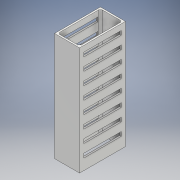
# Autodesk Inventor part: LiFeGuard
Saved by Autodesk Inventor 2018 (Build 220112000, 112)
## iProperties
Created: 2018-08-27
Part Number: LiFeGuard
Material: ABS プラスチック
Document SubType Name: Modeling
Designer: shun2
Density: 1.06 g/cm^3
Appearance: 滑らか - 白
Author: shun2
Autodesk Inventor part; units mm, degrees
ref_plane "YZ Plane" through (0, 0, 0) normal (1, 0, 0) x (0, 1, 0)
ref_plane "XZ Plane" through (0, 0, 0) normal (0, 1, 0) x (-1, 0, 0)
ref_plane "XY Plane" through (0, 0, 0) normal (0, 0, 1) x (1, 0, 0)
sketch "スケッチ1" plane through (0, 0, 0) normal (0, 0, 1) x (1, 0, 0)
  line L0 (0, 0) -> (30, 0)
  line L1 (30, 0) -> (30, 55)
  line L2 (30, 55) -> (0, 55)
  line L3 (0, 55) -> (0, 2)
  line L4 (2, 53) -> (2, 2)
  line L5 (2, 2) -> (28, 2)
  line L6 (28, 53) -> (28, 2)
  line L7 (2, 53) -> (28, 53)
  line L8 (0, 2) -> (0, 0)
  dimension "d0" = 30
  dimension "d1" = 55
  constraints: 18 end point, 5 perpendicular, 2 parallel, 1 horizontal, 1 vertical
  measures "d0" distance of L2.end L1.end
  measures "d1" distance of L1.end L0.end
extrude "押し出し1" add sketch "スケッチ1" along normal blind 130
sketch "スケッチ2" plane through (30, 0, 0) normal (1, 0, 0) x (0, 0, -1)
  line L0 (-130, 53) -> (-130, 2) projected
  line L1 (-123.1035, 50) -> (-118.1035, 50)
  line L2 (-118.1035, 50) -> (-118.1035, 5)
  line L3 (-118.1035, 5) -> (-123.1035, 5)
  line L4 (-123.1035, 5) -> (-123.1035, 50)
  line L5 (-108.1035, 50) -> (-103.1035, 50)
  line L6 (-103.1035, 50) -> (-103.1035, 5)
  line L7 (-103.1035, 5) -> (-108.1035, 5)
  line L8 (-108.1035, 5) -> (-108.1035, 50)
  line L9 (-93.1035, 50) -> (-88.1035, 50)
  line L10 (-88.1035, 50) -> (-88.1035, 5)
  line L11 (-88.1035, 5) -> (-93.1035, 5)
  line L12 (-93.1035, 5) -> (-93.1035, 50)
  line L13 (-78.1035, 50) -> (-73.1035, 50)
  line L14 (-73.1035, 50) -> (-73.1035, 5)
  line L15 (-73.1035, 5) -> (-78.1035, 5)
  line L16 (-78.1035, 5) -> (-78.1035, 50)
  line L17 (-63.1035, 50) -> (-58.1035, 50)
  line L18 (-58.1035, 50) -> (-58.1035, 5)
  line L19 (-58.1035, 5) -> (-63.1035, 5)
  line L20 (-63.1035, 5) -> (-63.1035, 50)
  line L21 (-48.1035, 50) -> (-43.1035, 50)
  line L22 (-43.1035, 50) -> (-43.1035, 5)
  line L23 (-43.1035, 5) -> (-48.1035, 5)
  line L24 (-48.1035, 5) -> (-48.1035, 50)
  line L25 (-33.1035, 50) -> (-28.1035, 50)
  line L26 (-28.1035, 50) -> (-28.1035, 5)
  line L27 (-28.1035, 5) -> (-33.1035, 5)
  line L28 (-33.1035, 5) -> (-33.1035, 50)
  line L29 (-18.1035, 50) -> (-13.1035, 50)
  line L30 (-13.1035, 50) -> (-13.1035, 5)
  line L31 (-13.1035, 5) -> (-18.1035, 5)
  line L32 (-18.1035, 5) -> (-18.1035, 50)
  line L33 (-123.1035, 50) -> (-118.1035, 50)
  line L34 (-108.1035, 50) -> (-103.1035, 50)
  line L35 (-93.1035, 50) -> (-88.1035, 50)
  line L36 (-78.1035, 50) -> (-73.1035, 50)
  line L37 (-63.1035, 50) -> (-58.1035, 50)
  line L38 (-48.1035, 50) -> (-43.1035, 50)
  line L39 (-33.1035, 50) -> (-28.1035, 50)
  line L40 (-18.1035, 50) -> (-13.1035, 50)
  line L41 (-18.1035, 5) -> (-13.1035, 5)
  line L42 (-33.1035, 5) -> (-28.1035, 5)
  line L43 (-48.1035, 5) -> (-43.1035, 5)
  line L44 (-63.1035, 5) -> (-58.1035, 5)
  line L45 (-78.1035, 5) -> (-73.1035, 5)
  line L46 (-93.1035, 5) -> (-88.1035, 5)
  line L47 (-123.1035, 5) -> (-118.1035, 5)
  line L48 (-108.1035, 5) -> (-103.1035, 5)
  point P0 (0, 0)
  point P1 (-44, 28.2547)
  dimension "d8" = 5
  dimension "d9" = 5
  dimension "d10" = 5
  dimension "d11" = 5
  dimension "d12" = 5
  dimension "d13" = 5
  dimension "d14" = 5
  dimension "d15" = 10
  dimension "d16" = 10
  dimension "d17" = 10
  dimension "d18" = 10
  dimension "d19" = 10
  dimension "d20" = 10
  dimension "d21" = 5
  dimension "d22" = 10
  constraints: 96 end point, 16 horizontal, 16 parallel, 8 perpendicular
  measures "d8" distance of L3.end L2.end
  measures "d9" distance of L6.end L7.end
  measures "d10" distance of L10.end L11.end
  measures "d11" distance of L14.end L15.end
  measures "d12" distance of L18.end L19.end
  measures "d13" distance of L22.end L23.end
  measures "d14" distance of L26.end L27.end
  measures "d15" distance between parallel lines of L8 L2
  measures "d16" distance between parallel lines of L12 L6
  measures "d17" distance between parallel lines of L16 L10
  measures "d18" distance between parallel lines of L20 L14
  measures "d19" distance between parallel lines of L24 L18
  measures "d20" distance between parallel lines of L28 L22
  measures "d21" distance of L30.end L31.end
  measures "d22" distance between parallel lines of L32 L26
extrude "押し出し2" cut sketch "スケッチ2" against normal blind 30
chamfer "面取り1" distance 2 angle 45 2 edges at (2, 53, 65) (28, 2, 65)
chamfer "面取り2" distance 2 angle 45 2 edges at (28, 53, 65) (2, 2, 65)
